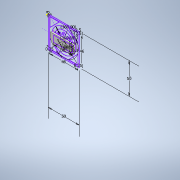
# Autodesk Inventor part: BaseCoilBrace
Saved by Autodesk Inventor 2022 (Build 260153000, 153)
## iProperties
Created: 2022-08-02
Part Number: BaseCoilBrace
Material: Generic
Document SubType Name: Modeling
Designer: sgioj
Density: 1 g/cm^3
Appearance: Default
Author: sgioj
Autodesk Inventor part; units mm, degrees
ref_plane "YZ Plane" through (0, 0, 0) normal (1, 0, 0) x (0, 1, 0)
ref_plane "XZ Plane" through (0, 0, 0) normal (0, 1, 0) x (-1, 0, 0)
ref_plane "XY Plane" through (0, 0, 0) normal (0, 0, 1) x (1, 0, 0)
sketch "Sketch1" plane through (0, 0, 0) normal (0, 0, 1) x (1, 0, 0)
  line L0 (0, 0) -> (50, 0)
  line L1 (50, 0) -> (50, -50)
  line L2 (50, -50) -> (0, -50)
  line L3 (0, -50) -> (0, 0)
  line L4 (2, -2) -> (48, -2)
  line L5 (48, -2) -> (48, -48)
  line L6 (48, -48) -> (2, -48)
  line L7 (2, -48) -> (2, -2)
  line L8 (2, -2) -> (48, -48) construction
  line L9 (48, -2) -> (2, -48) construction
  circle A0 centre (25, -25) radius 19.125
  circle A1 centre (25, -25) radius 14.75
  circle A2 centre (25, -25) radius 4.175
  circle A3 centre (31.678, -18.322) radius 2.45
  circle A4 centre (25, -15.5559) radius 2.45
  circle A5 centre (18.322, -18.322) radius 2.45
  circle A6 centre (15.5559, -25) radius 2.45
  circle A7 centre (18.322, -31.678) radius 2.45
  circle A8 centre (25, -34.4441) radius 2.45
  circle A9 centre (31.678, -31.678) radius 2.45
  circle A10 centre (34.4441, -25) radius 2.45
  line L10 (50, -25) -> (-10.9328, -25) construction
  line L11 (47.5, -2.5) -> (47.5, -17.5)
  line L12 (47.5, -2.5) -> (32.5, -2.5)
  line L13 (32.5, -2.5) -> (47.5, -17.5)
  line L14 (2.5, -17.5) -> (17.5, -2.5)
  line L15 (2.5, -2.5) -> (17.5, -2.5)
  line L16 (2.5, -2.5) -> (2.5, -17.5)
  line L17 (17.5, -47.5) -> (2.5, -32.5)
  line L18 (2.5, -47.5) -> (2.5, -32.5)
  line L19 (2.5, -47.5) -> (17.5, -47.5)
  line L20 (47.5, -32.5) -> (32.5, -47.5)
  line L21 (47.5, -47.5) -> (32.5, -47.5)
  line L22 (47.5, -47.5) -> (47.5, -32.5)
  line L23 (33.4104, -33.4104) -> (35.4298, -35.4298)
  line L24 (16.5896, -16.5896) -> (14.5702, -14.5702)
  line L25 (18.322, -20.772) -> (31.678, -20.772)
  line L26 (39.131, -20.772) -> (43.6518, -20.772)
  line L27 (39.131, -20.772) -> (31.678, -20.772)
  line L28 (18.322, -20.772) -> (10.869, -20.772)
  arc A11 (16.5896, -33.4104) -> (33.4104, -16.5896) centre (25, -25) ccw
  line L29 (10.869, -20.772) -> (6.3482, -20.772)
  arc A12 (16.5896, -16.5896) -> (16.5896, -33.4104) centre (25, -25) ccw
  line L30 (11.4766, -38.5234) -> (14.5702, -35.4298)
  line L31 (16.5896, -33.4104) -> (14.5702, -35.4298)
  line L32 (35.4298, -35.4298) -> (38.5234, -38.5234)
  line L33 (18.322, -31.678) -> (16.4147, -33.2318)
  line L34 (16.4147, -33.2318) -> (11.301, -38.3455)
  line L35 (31.678, -31.678) -> (33.5853, -33.2318)
  line L36 (33.5853, -33.2318) -> (38.699, -38.3455)
  dimension "d4" = 50
  dimension "d5" = 50
  dimension "d6" = 46
  dimension "d7" = 46
  dimension "d8" = 38.25
  dimension "d9" = 29.5
  dimension "d10" = 8.35
  dimension "d11" = 4.9
  dimension "d12" = 360
  dimension "d13" = 2
  dimension "d14" = 2
  dimension "d15" = 15
  dimension "d16" = 15
  dimension "d17" = 2.5
  dimension "d18" = 2.5
  dimension "d19" = 360
  dimension "d24" = 0.25
  dimension "d25" = 0.25
  constraints: 74 end point, 23 point on circle, 14 point on line, 11 centre point, 5 horizontal, 5 parallel, 3 coincident, 3 midpoint, 3 tangent, 2 perpendicular, 1 collinear, 1 vertical, 48 other
  measures "d4" distance of L1.end L2.end
  measures "d5" distance of L0.end L1.end
  measures "d6" distance of L5.end L6.end
  measures "d7" distance of L4.end L5.end
  measures "d8" diameter of A0
  measures "d9" diameter of A1
  measures "d10" diameter of A2
  measures "d11" diameter of A3
  measures "d13" distance between parallel lines of L3 L7
  measures "d14" distance between parallel lines of L0 L4
  measures "d15" distance of L11.start L11.end
  measures "d16" distance of L11.start L12.end
  measures "d17" horizontal distance of L11.start L0.end
  measures "d18" distance from line of L1 L11.start
  measures "d24" distance from line of L9 L33.end
  measures "d25" distance from line of L8 L35.end
extrude "Extrusion1" add sketch "Sketch1" along normal blind 2.7 contours A0 L36 A1 L26 | L29 A1 L34 A0 | A1 L36 A11 L27 | L28 A12 L34 A1 | A6 | A8 | A10 | A11 L35 A9 A7 L33 A12 L28 L25 L27 | A11 A9 L35 | A9 | L33 A7 A12 | A7 | A2
extrude "Extrusion2" add sketch "Sketch1" against normal blind 1.8 contours A0 L36 A1 L26 | A0 L32 A1 L36 | L29 A1 L34 A0 | L34 A1 L30 A0
sketch "Sketch2" plane through (0, 0, 2.7) normal (0, 0, 1) x (1, 0, 0)
  line L0 (11.3606, -22.3794) -> (41.3606, -22.3794)
  line L1 (41.3606, -22.3794) -> (41.3606, -32.6794)
  line L2 (41.3606, -32.6794) -> (11.3606, -32.6794)
  line L3 (11.3606, -32.6794) -> (11.3606, -22.3794)
  point P0 (0, 0)
  dimension "d26" = 30
  dimension "d27" = 10.3
  constraints: 8 end point, 2 parallel, 1 horizontal, 1 perpendicular
  measures "d26" distance of L1.end L2.end
  measures "d27" distance of L0.end L1.end
body "Solid1"
